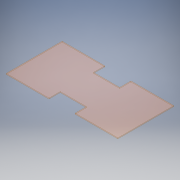
# Autodesk Inventor part: EBoard
Saved by Autodesk Inventor 2019 (Build 230136000, 136)
## iProperties
Created: 2018-02-22
Part Number: EBoard
Material: Polycarbonate, Clear
Document SubType Name: Modeling
Designer: james
Density: 1.2 g/cm^3
Appearance: Clear - Light(1)
Mass: 971.548 g
Surface Area: 3500.4 cm^2
Volume: 809.623 cm^3
Author: james
Autodesk Inventor part; units mm, degrees
ref_plane "YZ Plane" through (0, 0, 0) normal (1, 0, 0) x (0, 1, 0)
ref_plane "XZ Plane" through (0, 0, 0) normal (0, 1, 0) x (-1, 0, 0)
ref_plane "XY Plane" through (0, 0, 0) normal (0, 0, 1) x (1, 0, 0)
sketch "Sketch1" plane through (0, 0, 0) normal (0, 1, 0) x (-1, 0, 0)
  line L0 (171.4161, 216.9837) -> (-425.4839, 216.9837)
  line L1 (-425.4839, 216.9837) -> (-425.4839, -100.5163)
  line L2 (-425.4839, -100.5163) -> (171.4161, -100.5163)
  line L3 (171.4161, -100.5163) -> (171.4161, 216.9837)
  point P0 (0, 0)
  dimension "d0" = 317.5
  dimension "d1" = 596.9
  constraints: 8 end point, 2 parallel, 1 horizontal, 1 perpendicular
  measures "d0" distance of L2.end L0.start
  measures "d1" distance of L1.end L2.end
extrude "Extrusion1" add sketch "Sketch1" along normal blind 4.7625
sketch "Sketch2" plane through (0, 4.7625, 0) normal (0, 1, 0) x (1, 0, 0)
  line L0 (57.1839, 30.6663) -> (196.8839, 30.6663)
  line L1 (196.8839, 30.6663) -> (196.8839, 100.5163)
  line L2 (196.8839, 100.5163) -> (57.1839, 100.5163)
  line L3 (57.1839, 100.5163) -> (57.1839, 30.6663)
  line L4 (57.1839, -147.1337) -> (196.8839, -147.1337)
  line L5 (196.8839, -147.1337) -> (196.8839, -216.9837)
  line L6 (196.8839, -216.9837) -> (57.1839, -216.9837)
  line L7 (57.1839, -216.9837) -> (57.1839, -147.1337)
  line L8 (425.4839, -216.9837) -> (425.4839, 100.5163) projected
  line L9 (-171.4161, 100.5163) -> (-171.4161, -216.9837) projected
  line L10 (-171.4161, -216.9837) -> (425.4839, -216.9837) projected
  line L11 (425.4839, 100.5163) -> (-171.4161, 100.5163) projected
  point P0 (0, 0)
  dimension "d4" = 0
  dimension "d5" = 228.6
  dimension "d6" = 0
  dimension "d7" = 228.6
  dimension "d8" = 0
  dimension "d9" = 0
  dimension "d10" = 69.85
  dimension "d11" = 69.85
  constraints: 16 end point, 4 parallel, 2 horizontal, 2 perpendicular
  measures "d4" distance between parallel lines of L5 L1
  measures "d5" distance between parallel lines of L8 L5
  measures "d6" distance between parallel lines of L3 L7
  measures "d7" distance between parallel lines of L9 L3
  measures "d8" distance between parallel lines of L10 L6
  measures "d9" distance between parallel lines of L11 L2
  measures "d10" distance between parallel lines of L11 L0
  measures "d11" distance between parallel lines of L10 L4
extrude "Extrusion2" cut sketch "Sketch2" along normal mid plane 25.4 contours L3 L2 L1 L0 | L7 L4 L5 L6
sketch "Sketch3" plane through (0, 4.7625, 0) normal (0, 1, 0) x (1, 0, 0)
  line L0 (-203.1439, 127.0873) -> (472.3707, 127.0873)
  line L1 (472.3707, 127.0873) -> (472.3707, 90.9913)
  line L2 (472.3707, 90.9913) -> (-203.1439, 90.9913)
  line L3 (-203.1439, 90.9913) -> (-203.1439, 127.0873)
  line L4 (463.6684, -207.4587) -> (-190.0904, -207.4587)
  line L5 (-190.0904, -207.4587) -> (-190.0904, -244.0242)
  line L6 (-190.0904, -244.0242) -> (463.6684, -244.0242)
  line L7 (463.6684, -244.0242) -> (463.6684, -207.4587)
  line L8 (425.4839, 100.5163) -> (196.8839, 100.5163) projected
  line L9 (196.8839, -216.9837) -> (425.4839, -216.9837) projected
  point P0 (0, 0)
  dimension "d14" = 9.525
  dimension "d15" = 9.525
  constraints: 16 end point, 4 parallel, 2 horizontal, 2 perpendicular
  measures "d14" distance between parallel lines of L2 L8
  measures "d15" distance between parallel lines of L9 L4
extrude "Extrusion3" cut sketch "Sketch3" against normal blind 25.4
body "Solid1"
